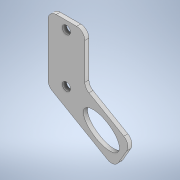
# Autodesk Inventor part: base
Saved by Autodesk Inventor 2022 (Build 260153000, 153)
## iProperties
Created: 2022-10-14
Part Number: base
Material: Generic
Document SubType Name: Modeling
Designer: Usuario
Density: 1 g/cm^3
Appearance: Default
Author: Usuario
Autodesk Inventor part; units mm, degrees
ref_plane "YZ Plane" through (0, 0, 0) normal (1, 0, 0) x (0, 1, 0)
ref_plane "XZ Plane" through (0, 0, 0) normal (0, 1, 0) x (-1, 0, 0)
ref_plane "XY Plane" through (0, 0, 0) normal (0, 0, 1) x (1, 0, 0)
sketch "Sketch1" plane through (0, 0, 0) normal (0, 0, 1) x (1, 0, 0)
  line L0 (-12.4598, 60) -> (12.4598, 60)
  line L1 (-22.4598, -14.4802) -> (-22.4598, 50)
  arc A0 (-12.4598, 60) -> (-22.4598, 50) centre (-12.4598, 50) ccw
  arc A1 (22.4598, 50) -> (12.4598, 60) centre (12.4598, 50) ccw
  line L2 (27.4598, -2.8868) -> (70.0912, -27.5)
  line L3 (22.4598, 0) -> (71.6863, 0) construction
  line L4 (73.7514, -41.1603) -> (63.7514, -58.4808)
  line L5 (50.0912, -62.141) -> (-17.4598, -23.1405)
  line L6 (22.4598, 50) -> (22.4598, 5.7735)
  arc A2 (-22.4598, -14.4802) -> (-17.4598, -23.1405) centre (-12.4598, -14.4802) ccw
  arc A3 (22.4598, 5.7735) -> (27.4598, -2.8868) centre (32.4598, 5.7735) ccw
  arc A4 (73.7514, -41.1603) -> (70.0912, -27.5) centre (65.0912, -36.1603) ccw
  arc A5 (50.0912, -62.141) -> (63.7514, -58.4808) centre (55.0912, -53.4808) ccw
  point P0 (0, 0)
  point P1 (0, 60)
  point P2 (78.7514, -32.5)
  point P3 (58.7514, -67.141)
  dimension "d0" = 10
  dimension "d11" = 65
  dimension "d12" = 30
  dimension "d13" = 40
  dimension "d14" = 10
  constraints: 14 end point, 12 point on circle, 12 tangent, 6 centre point, 6 point on line, 4 equal radius, 3 perpendicular, 2 horizontal, 1 equal length, 1 horizontal alignment, 1 midpoint, 1 parallel, 1 vertical alignment
  measures "d0" radius of A0
  measures "d11" distance of L3.start point (78.751, -32.5)
  measures "d12" angle of L2 L3
  measures "d13" distance of point (78.751, -32.5) point (58.751, -67.141)
  measures "d14" radius of A2
extrude "Extrusion1" add sketch "Sketch1" along normal blind 5
sketch "Sketch2" plane through (0, 0, 5) normal (0, 0, 1) x (1, 0, 0)
  circle A0 centre (0, 50) radius 5
  line L0 (-22.4598, 50) -> (-22.4598, -14.4802) construction
  line L1 (-22.4598, 17.7599) -> (22.4598, 27.8868) construction
  line L2 (22.4598, 5.7735) -> (22.4598, 50) construction
  line L3 (12.4598, 60) -> (-12.4598, 60) projected
  circle A1 centre (0, -10) radius 5
  line L4 (63.7514, -58.4808) -> (73.7514, -41.1603) projected
  ellipse E0 centre (42.7707, -34.8205) end of major axis (63.7179, -46.9144) minor radius 13.5207
  line L5 (70.0912, -27.5) -> (27.4598, -2.8868) projected
  point P0 (0, 0)
  point P1 (0, 22.8233)
  dimension "d5" = 10
  dimension "d7" = 10
  dimension "d15" = 10
  dimension "d16" = 10
  dimension "d19" = 30
  dimension "d20" = 20
  constraints: 3 centre point, 3 midpoint, 2 end point, 2 vertical alignment
  measures "d5" diameter of A0
  measures "d7" distance from line of L3 A0.centre
  measures "d15" diameter of A1
  measures "d16" distance of point (0, 0) A1.centre
  measures "d19" distance from line of L4 E0.centre
  measures "d20" distance from line of L5 E0.centre
extrude "Extrusion2" cut sketch "Sketch2" against normal up to surface (5 mm away)
body "Solid1"
